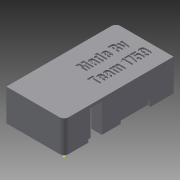
# Autodesk Inventor part: Negative Cap 545
Saved by Autodesk Inventor 2015 (Build 190159000, 159)
## iProperties
Created: 2015-01-23
Part Number: Negative Cap 545
Material: Generic
Document SubType Name: Modeling
Designer: pltwe4
Density: 1 g/cm^3
Appearance: Default
Author: pltwe4
Autodesk Inventor part; units mm, degrees
ref_plane "YZ Plane" through (0, 0, 0) normal (1, 0, 0) x (0, 1, 0)
ref_plane "XZ Plane" through (0, 0, 0) normal (0, 1, 0) x (-1, 0, 0)
ref_plane "XY Plane" through (0, 0, 0) normal (0, 0, 1) x (1, 0, 0)
sketch "Sketch1" plane through (0, 0, 0) normal (0, 1, 0) x (-1, 0, 0)
  line L0 (0, 0) -> (24.5364, 0)
  line L1 (24.5364, 0) -> (24.5364, -46.5582)
  line L2 (24.5364, -46.5582) -> (0, -46.5582)
  line L3 (0, -46.5582) -> (0, 0)
  dimension "d0" = 46.5582
  dimension "d1" = 24.5364
  constraints: 8 end point, 2 parallel, 1 horizontal, 1 perpendicular
  measures "d0" distance of L0.end L1.end
  measures "d1" distance of L1.end L2.end
extrude "Extrusion1" add sketch "Sketch1" along normal blind 13.5382
sketch "Sketch2" plane through (0, 0, 0) normal (0, -1, 0) x (1, 0, 0)
  point P0 (0, 0)
fillet "Fillet1" radius 1.905 1 edges at (-24.5364, 6.7691, -46.5582)
fillet "Fillet2" radius 1.905 1 edges at (0, 6.7691, 0)
sketch "Sketch3" plane through (0, 0, 0) normal (0, -1, 0) x (1, 0, 0)
  line L0 (-1.905, 0) -> (-24.5364, 0) projected
  arc A0 (0, -1.905) -> (-1.905, 0) centre (-1.905, -1.905) ccw projected
  line L1 (0, -46.5582) -> (0, -1.905) projected
  line L2 (-22.6314, -46.5582) -> (0, -46.5582) projected
  arc A1 (-24.5364, -44.6532) -> (-22.6314, -46.5582) centre (-22.6314, -44.6532) ccw projected
  line L3 (-24.5364, 0) -> (-24.5364, -44.6532) projected
  line L4 (-2.54, -2.54) -> (-21.9964, -2.54)
  line L5 (-21.9964, -44.0182) -> (-2.54, -44.0182)
  line L6 (0, -12.9032) -> (-4.445, -12.9032)
  line L7 (-4.445, -16.0782) -> (0, -16.0782)
  line L8 (-2.54, -44.0182) -> (-2.54, -18.6182)
  line L9 (-2.54, -10.3632) -> (-2.54, -2.54)
  line L10 (-4.445, -12.9032) -> (-4.445, -10.3632)
  line L11 (-4.445, -10.3632) -> (-2.54, -10.3632)
  line L12 (-4.445, -16.0782) -> (-4.445, -18.6182)
  line L13 (-4.445, -18.6182) -> (-2.54, -18.6182)
  line L14 (-21.9964, -10.3632) -> (-18.4404, -10.3632)
  line L15 (-18.4404, -10.3632) -> (-18.4404, -18.6182)
  line L16 (-18.4404, -18.6182) -> (-21.9964, -18.6182)
  line L17 (-21.9964, -2.54) -> (-21.9964, -10.3632)
  line L18 (-21.9964, -18.6182) -> (-21.9964, -44.0182)
  line L19 (0, -14.4907) -> (-5.2569, -14.4907) construction
  line L20 (-4.445, -11.6332) -> (-18.4404, -11.6332)
  line L21 (-4.445, -17.3482) -> (-18.4404, -17.3482)
  point P0 (0, 0)
  dimension "d7" = 2.54
  dimension "d9" = 2.54
  dimension "d11" = 3.175
  dimension "d13" = 4.445
  dimension "d14" = 2.54
  dimension "d15" = 2.54
  dimension "d16" = 2.54
  dimension "d17" = 2.54
  dimension "d20" = 2.54
  dimension "d21" = 6.096
  dimension "d22" = 2.54
  dimension "d37" = 32.0675
  constraints: 36 end point, 9 perpendicular, 7 parallel, 5 point on line, 4 horizontal, 2 collinear, 2 midpoint, 2 vertical, 1 other
  measures "d7" distance between parallel lines of L0 L4
  measures "d9" distance between parallel lines of L2 L5
  measures "d11" distance between parallel lines of L6 L7
  measures "d13" distance between parallel lines of L1 L10
  measures "d14" distance of L7.start L12.end
  measures "d15" distance of L6.end L10.end
  measures "d16" distance between parallel lines of L1 L8
  measures "d17" distance between parallel lines of L1 L9
  measures "d20" distance between parallel lines of L3 L18
  measures "d21" distance between parallel lines of L3 L15
  measures "d22" distance between parallel lines of L3 L17
  measures "d37" distance between parallel lines of L2 L19
extrude "Extrusion2" cut sketch "Sketch3" against normal blind 12.2682 contours L1 L7 L12 L21 L15 L20 L10 L6 | L20 L15 L14 L17 L4 L9 L11 L10 | L12 L13 L8 L5 L18 L16 L15 L21
sketch "Sketch4" plane through (0, 12.2682, 0) normal (0, -1, 0) x (1, 0, 0)
  line L0 (-4.3434, -23.6982) -> (-17.0434, -23.6982)
  line L1 (-17.0434, -23.6982) -> (-17.0434, -35.1282)
  line L2 (-17.0434, -35.1282) -> (-4.3434, -35.1282)
  line L3 (-4.3434, -35.1282) -> (-4.3434, -23.6982)
  line L4 (-2.54, -44.0182) -> (-21.9964, -44.0182) projected
  line L5 (-2.54, -18.6182) -> (-2.54, -44.0182) projected
  line L6 (-10.6934, -23.6982) -> (-10.6934, -35.1282) construction
  line L7 (-24.5364, 0) -> (-24.5364, -44.6532) construction
  line L8 (-22.6314, -46.5582) -> (0, -46.5582) construction
  point P0 (0, 0)
  dimension "d23" = 13.843
  dimension "d24" = 12.7
  dimension "d25" = 11.43
  dimension "d26" = 22.86
  constraints: 10 end point, 2 midpoint, 2 parallel, 1 horizontal, 1 perpendicular
  measures "d23" distance between parallel lines of L7 L6
  measures "d24" distance between parallel lines of L1 L3
  measures "d25" distance between parallel lines of L0 L2
  measures "d26" distance between parallel lines of L8 L0
extrude "Extrusion3" add sketch "Sketch4" along normal up to surface (12.2682 mm away)
sketch "Sketch5" plane through (-4.3434, 12.2682, -35.1282) normal (0, 0, -1) x (-1, 0, 0)
  line L0 (0, 0) -> (0, -12.2682) projected
  line L1 (12.7, 0) -> (12.7, -12.2682) projected
  line L2 (12.7, -12.2682) -> (0, -12.2682) projected
  arc A0 (8.2396, -6.5778) -> (4.4604, -6.5778) centre (6.35, -5.1816) ccw
  line L3 (6.35, -12.2682) -> (6.35, 0) construction
  line L4 (17.653, 0) -> (-1.8034, 0) construction
  line L5 (8.2396, -6.5778) -> (8.4707, -7.62)
  line L6 (8.4707, -7.62) -> (11.0107, -7.62)
  line L7 (11.0107, -7.62) -> (12.7, 0)
  line L8 (4.4604, -6.5778) -> (4.2293, -7.62)
  line L9 (4.2293, -7.62) -> (1.6893, -7.62)
  line L10 (1.6893, -7.62) -> (0, 0)
  point P0 (-4.3434, -12.2682)
  dimension "d29" = 7.0866
  dimension "d30" = 4.699
  dimension "d32" = 7.62
  dimension "d33" = 2.54
  dimension "d36" = 25
  constraints: 14 end point, 2 horizontal, 2 point on circle, 2 point on line, 1 centre point, 1 equal length, 1 midpoint, 1 parallel, 1 vertical, 2 other
  measures "d29" distance from line of L2 A0.centre
  measures "d30" diameter of A0
  measures "d32" distance between parallel lines of L4 L6
  measures "d33" distance of L5.end L6.end
  measures "d36" angle of L5 L8
extrude "Extrusion4" cut sketch "Sketch5" against normal up to surface (11.43 mm away)
sketch "Sketch6" plane through (0, 12.2682, 0) normal (0, -1, 0) x (1, 0, 0)
  line L0 (-4.445, -10.3632) -> (-4.445, -12.9032) projected
  line L1 (-4.445, -16.0782) -> (-4.445, -18.6182) projected
  line L2 (-18.4404, -18.6182) -> (-18.4404, -10.3632) projected
  line L3 (0, -12.9032) -> (0, -16.0782) projected
  line L4 (0, -16.0782) -> (-4.445, -16.0782) projected
  line L5 (-4.445, -12.9032) -> (0, -12.9032) projected
  line L6 (-4.445, -10.3632) -> (-18.4404, -10.3632)
  line L7 (-18.4404, -18.6182) -> (-4.445, -18.6182)
  line L8 (-1.27, -12.9032) -> (-1.27, -16.0782)
  point P0 (0, 0)
  dimension "d46" = 1.27
  constraints: 6 end point, 2 point on line, 1 horizontal, 1 parallel, 1 perpendicular
  measures "d46" distance between parallel lines of L8 L3
extrude "Extrusion5" cut sketch "Sketch6" against normal blind 0.635
sketch "Sketch7" plane through (0, 0, 0) normal (0, -1, 0) x (1, 0, 0)
  line L0 (0, -12.9032) -> (0, -1.905) projected
  line L1 (0, -1.905) -> (0, -46.5582) projected
  line L2 (0, -10.3632) -> (-0.635, -10.3632)
  line L3 (-1.27, -10.9982) -> (-1.27, -12.2682)
  arc A0 (-0.635, -10.3632) -> (-1.27, -10.9982) centre (-0.635, -10.9982) ccw
  line L4 (-1.905, -12.9032) -> (-4.445, -12.9032)
  line L5 (-4.445, -10.3632) -> (-4.445, -12.9032) projected
  arc A1 (-1.905, -12.9032) -> (-1.27, -12.2682) centre (-1.905, -12.2682) ccw
  line L6 (0, -10.3632) -> (0, -12.9032)
  line L7 (0, -12.9032) -> (-1.905, -12.9032)
  line L8 (-4.445, -12.9032) -> (0, -12.9032) projected
  point P0 (0, 0)
  point P1 (-1.27, -10.3632)
  point P2 (-1.27, -12.9032)
  dimension "d40" = 1.27
  dimension "d41" = 2.54
  dimension "d42" = 0.635
  dimension "d43" = 0.635
  constraints: 10 end point, 5 point on line, 5 tangent, 4 point on circle, 2 centre point, 2 collinear, 2 perpendicular, 1 parallel
  measures "d40" distance of L2.start point (-1.27, -10.363)
  measures "d41" distance of point (-1.27, -10.363) point (-1.27, -12.903)
  measures "d42" radius of A0
  measures "d43" radius of A1
extrude "Extrusion7" add sketch "Sketch6" against normal blind 0.635 contours L5 L3 L4 L8
extrude "Extrusion8" cut sketch "Sketch7" against normal up to surface (12.2682 mm away)
sketch "Sketch8" plane through (0, 0, -46.5582) normal (1, 0, 0) x (0, 0, -1)
  line L0 (-36.195, 0) -> (-36.195, 12.2682) projected
  line L1 (-30.48, 12.2682) -> (-36.195, 12.2682) projected
  line L2 (-30.48, 12.2682) -> (-30.48, 0) projected
  line L3 (0, 0) -> (-30.48, 0) projected
  line L4 (0, 0) -> (0, 13.5382) projected
  line L5 (-44.6532, 13.5382) -> (0, 13.5382) projected
  line L6 (-44.6532, 0) -> (-44.6532, 13.5382) projected
  line L7 (-36.195, 0) -> (-44.6532, 0) projected
  line L8 (-22.5397, 0) -> (-22.5397, 2.54)
  line L9 (-22.5397, 2.54) -> (-9.8397, 2.54)
  line L10 (-9.8397, 2.54) -> (-9.8397, 0)
  point P0 (-46.5582, 0)
  dimension "d51" = 2.54
  dimension "d52" = 12.7
  constraints: 6 end point, 2 perpendicular, 2 point on line, 1 vertical
  measures "d51" distance of L9.end L10.end
  measures "d52" distance of L8.end L9.end
extrude "Extrusion9" cut sketch "Sketch8" against normal blind 1.27 contours L8 L9 L10 L3
sketch "Sketch9" plane through (-4.3434, 12.2682, -35.1282) normal (0, 0, -1) x (-1, 0, 0)
  line L0 (12.7, 0) -> (11.0107, -7.62) projected
  line L1 (11.0107, -7.62) -> (8.4707, -7.62) projected
  line L2 (8.4707, -7.62) -> (8.2396, -6.5778) projected
  arc A0 (8.2396, -6.5778) -> (4.4604, -6.5778) centre (6.35, -5.1816) ccw projected
  line L3 (4.4604, -6.5778) -> (4.2293, -7.62) projected
  line L4 (4.2293, -7.62) -> (1.6893, -7.62) projected
  line L5 (1.6893, -7.62) -> (0, 0) projected
  line L6 (12.7, 0) -> (0, 0) projected
  line L7 (1.6893, -7.62) -> (11.0107, -7.62)
  line L8 (4.2293, -7.62) -> (1.6893, -7.62) projected
  point P0 (-4.3434, -12.2682)
  constraints: 2 end point, 1 collinear
extrude "Extrusion10" add sketch "Sketch9" along normal blind 2.54
sketch "Sketch10" plane through (0, 13.5382, 0) normal (0, 1, 0) x (1, 0, 0)
  arc A0 (-1.905, 0) -> (0, 1.905) centre (-1.905, 1.905) ccw projected
  line L0 (0, 1.905) -> (0, 46.5582) projected
  line L1 (0, 46.5582) -> (-22.6314, 46.5582) projected
  arc A1 (-22.6314, 46.5582) -> (-24.5364, 44.6532) centre (-22.6314, 44.6532) ccw projected
  line L2 (-24.5364, 44.6532) -> (-24.5364, 0) projected
  line L3 (-24.5364, 0) -> (-1.905, 0) projected
  line L4 (-17.6657, 19.1516) -> (-17.6657, 44.5516) construction
  line L5 (-17.6657, 44.5516) -> (-4.9657, 44.5516) construction
  line L6 (-4.9657, 44.5516) -> (-4.9657, 19.1516) construction
  line L7 (-4.9657, 19.1516) -> (-17.6657, 19.1516) construction
  line L8 (-17.6657, 31.8516) -> (-4.9657, 31.8516) construction
  line L9 (-24.5364, 0) -> (-24.5364, 44.6532) construction
  line L10 (-24.5364, 22.3266) -> (0, 22.3266) construction
  line L11 (-11.3157, 19.1516) -> (-11.3157, 44.5516) construction
  line L12 (-22.6314, 46.5582) -> (0, 46.5582) construction
  line L13 (-11.3157, 46.5582) -> (-11.3157, 0) construction
  line L14 (-17.6657, 25.993) -> (-13.2207, 25.993)
  line L15 (-13.2207, 25.993) -> (-13.2207, 24.9814)
  line L16 (-13.2207, 24.9814) -> (-16.222, 24.9814)
  line L17 (-16.222, 24.9814) -> (-13.2207, 24.5761)
  line L18 (-13.2207, 24.5761) -> (-13.2207, 23.8627)
  line L19 (-13.2207, 23.8627) -> (-16.155, 23.4406)
  line L20 (-16.155, 23.4406) -> (-13.2207, 23.4373)
  line L21 (-13.2207, 23.4373) -> (-13.2207, 22.4257)
  line L22 (-13.2207, 22.4257) -> (-17.6657, 22.4257)
  line L23 (-17.6657, 22.4257) -> (-17.6657, 23.923)
  spline S0 degree 2 poles (-17.6657, 23.923) (-17.2671, 23.9866) (-16.7211, 24.0603) knots 0 0 0 1 1 1
  line L24 (-16.7211, 24.0603) -> (-15.5889, 24.2244)
  line L25 (-15.5889, 24.2244) -> (-17.6657, 24.4857)
  line L26 (-17.6657, 24.4857) -> (-17.6657, 25.993)
  line L27 (-15.4549, 27.4166) -> (-15.4549, 26.3749)
  line L28 (-15.4549, 26.3749) -> (-15.6994, 26.3749)
  spline S1 degree 2 poles (-15.6994, 26.3749) (-16.1215, 26.3749) (-16.5804, 26.5692) (-16.9321, 27.1587) (-16.9321, 27.6277) knots 0 0 0 1 2 3 3 3
  spline S2 degree 2 poles (-16.9321, 27.6277) (-16.9321, 28.1904) (-16.5335, 28.7632) (-15.954, 28.8771) (-15.0496, 28.8771) knots 0 0 0 1 2 3 3 3
  line L29 (-15.0496, 28.8771) -> (-13.2207, 28.8771)
  line L30 (-13.2207, 28.8771) -> (-13.2207, 27.7985)
  line L31 (-13.2207, 27.7985) -> (-13.5456, 27.7985)
  spline S3 degree 2 poles (-13.5456, 27.7985) (-13.3513, 27.698) (-13.1537, 27.3765) (-13.1537, 27.152) knots 0 0 0 1 2 2 2
  spline S4 degree 2 poles (-13.1537, 27.152) (-13.1537, 26.8606) (-13.482, 26.3749) (-14.0347, 26.3749) knots 0 0 0 1 2 2 2
  line L32 (-14.0347, 26.3749) -> (-14.3328, 26.3749)
  spline S5 degree 2 poles (-14.3328, 26.3749) (-14.7414, 26.3749) (-15.0396, 26.6328) (-15.2372, 27.1453) knots 0 0 0 1 2 2 2
  spline S6 degree 2 poles (-15.2372, 27.1453) (-15.4516, 27.6913) (-15.599, 27.7684) (-15.8267, 27.7684) knots 0 0 0 1 2 2 2
  spline S7 degree 2 poles (-15.8267, 27.7684) (-16.1115, 27.7684) (-16.2856, 27.6846) (-16.2856, 27.5841) knots 0 0 0 1 2 2 2
  spline S8 degree 2 poles (-16.2856, 27.5841) (-16.2856, 27.4702) (-16.1416, 27.4166) (-15.8368, 27.4166) knots 0 0 0 1 2 2 2
  line L33 (-15.8368, 27.4166) -> (-15.4549, 27.4166)
  spline S9 degree 2 poles (-14.9558, 27.7684) (-14.7615, 27.5004) (-14.4969, 27.4166) (-14.249, 27.4166) knots 0 0 0 1 2 2 2
  spline S10 degree 2 poles (-14.249, 27.4166) (-13.9643, 27.4166) (-13.8002, 27.4903) (-13.8002, 27.6009) knots 0 0 0 1 2 2 2
  spline S11 degree 2 poles (-13.8002, 27.6009) (-13.8002, 27.7047) (-13.9308, 27.7684) (-14.2055, 27.7684) knots 0 0 0 1 2 2 2
  line L34 (-14.2055, 27.7684) -> (-14.9558, 27.7684)
  line L35 (-17.6657, 31.7813) -> (-13.2207, 31.7813)
  line L36 (-13.2207, 31.7813) -> (-13.2207, 30.6725)
  line L37 (-13.2207, 30.6725) -> (-13.4853, 30.6725)
  spline S12 degree 2 poles (-13.4853, 30.6725) (-13.3178, 30.5117) (-13.1537, 30.1634) (-13.1537, 29.9691) knots 0 0 0 1 2 2 2
  spline S13 degree 2 poles (-13.1537, 29.9691) (-13.1537, 29.7112) (-13.425, 29.3327) (-13.7834, 29.2255) (-14.1854, 29.2255) knots 0 0 0 1 2 3 3 3
  line L38 (-14.1854, 29.2255) -> (-15.8937, 29.2255)
  spline S14 degree 2 poles (-15.8937, 29.2255) (-16.3124, 29.2255) (-16.6642, 29.3327) (-16.9321, 29.7179) (-16.9321, 29.9825) knots 0 0 0 1 2 3 3 3
  spline S15 degree 2 poles (-16.9321, 29.9825) (-16.9321, 30.1902) (-16.7847, 30.5318) (-16.634, 30.6725) knots 0 0 0 1 2 2 2
  line L39 (-16.634, 30.6725) -> (-17.6657, 30.6725)
  line L40 (-17.6657, 30.6725) -> (-17.6657, 31.7813)
  spline S16 degree 2 poles (-15.9473, 30.6725) (-16.1483, 30.6725) (-16.2856, 30.6022) (-16.2856, 30.5017) knots 0 0 0 1 2 2 2
  spline S17 degree 2 poles (-16.2856, 30.5017) (-16.2856, 30.4045) (-16.1617, 30.3342) (-15.9473, 30.3342) knots 0 0 0 1 2 2 2
  line L41 (-15.9473, 30.3342) -> (-14.162, 30.3342)
  spline S18 degree 2 poles (-14.162, 30.3342) (-13.9409, 30.3342) (-13.8002, 30.4012) (-13.8002, 30.495) knots 0 0 0 1 2 2 2
  spline S19 degree 2 poles (-13.8002, 30.495) (-13.8002, 30.6022) (-13.9576, 30.6725) (-14.2624, 30.6725) knots 0 0 0 1 2 2 2
  line L42 (-14.2624, 30.6725) -> (-15.9473, 30.6725)
  line L43 (-14.9793, 34.6921) -> (-14.9793, 33.2551)
  line L44 (-14.9793, 33.2551) -> (-14.1921, 33.2551)
  spline S20 degree 2 poles (-14.1921, 33.2551) (-13.9442, 33.2551) (-13.8002, 33.3255) (-13.8002, 33.4293) knots 0 0 0 1 2 2 2
  spline S21 degree 2 poles (-13.8002, 33.4293) (-13.8002, 33.5566) (-13.9911, 33.6403) (-14.2624, 33.6403) knots 0 0 0 1 2 2 2
  line L45 (-14.2624, 33.6403) -> (-14.7414, 33.6403)
  line L46 (-14.7414, 33.6403) -> (-14.7414, 34.6921)
  line L47 (-14.7414, 34.6921) -> (-14.4735, 34.6921)
  spline S22 degree 2 poles (-14.4735, 34.6921) (-14.1352, 34.6921) (-13.7734, 34.6084) (-13.3614, 34.2935) (-13.1537, 33.8145) (-13.1537, 33.4494) knots 0 0 0 1 2 3 4 4 4
  spline S23 degree 2 poles (-13.1537, 33.4494) (-13.1537, 33.0977) (-13.358, 32.5617) (-13.7131, 32.2603) (-14.1385, 32.1464) (-14.5438, 32.1464) knots 0 0 0 1 2 3 4 4 4
  line L48 (-14.5438, 32.1464) -> (-15.609, 32.1464)
  spline S24 degree 2 poles (-15.609, 32.1464) (-16.0847, 32.1464) (-16.6374, 32.4043) (-16.9321, 32.9938) (-16.9321, 33.3723) knots 0 0 0 1 2 3 3 3
  spline S25 degree 2 poles (-16.9321, 33.3723) (-16.9321, 33.8413) (-16.5771, 34.4476) (-15.9942, 34.6921) (-15.4616, 34.6921) knots 0 0 0 1 2 3 3 3
  line L49 (-15.4616, 34.6921) -> (-14.9793, 34.6921)
  line L50 (-15.5722, 33.58) -> (-15.8368, 33.58)
  spline S26 degree 2 poles (-15.8368, 33.58) (-16.1215, 33.58) (-16.2856, 33.5197) (-16.2856, 33.4259) knots 0 0 0 1 2 2 2
  spline S27 degree 2 poles (-16.2856, 33.4259) (-16.2856, 33.3087) (-16.145, 33.2551) (-15.8368, 33.2551) knots 0 0 0 1 2 2 2
  line L51 (-15.8368, 33.2551) -> (-15.5722, 33.2551)
  line L52 (-15.5722, 33.2551) -> (-15.5722, 33.58)
  line L53 (-17.6657, 36.0789) -> (-17.6657, 37.2312)
  spline S28 degree 2 poles (-17.6657, 37.2312) (-17.6657, 37.7805) (-17.4949, 38.3432) (-16.9757, 38.6883) (-16.3995, 38.6883) knots 0 0 0 1 2 3 3 3
  spline S29 degree 2 poles (-16.3995, 38.6883) (-16.011, 38.6883) (-15.7028, 38.4437) (-15.6224, 38.082) knots 0 0 0 1 2 2 2
  spline S30 degree 2 poles (-15.6224, 38.082) (-15.5286, 38.4839) (-15.1099, 38.7686) (-14.6745, 38.7686) knots 0 0 0 1 2 2 2
  line L54 (-14.6745, 38.7686) -> (-14.2658, 38.7686)
  spline S31 degree 2 poles (-14.2658, 38.7686) (-13.8136, 38.7686) (-13.3815, 38.5643) (-13.2207, 38.1121) (-13.2207, 37.4154) knots 0 0 0 1 2 3 3 3
  line L55 (-13.2207, 37.4154) -> (-13.2207, 36.0789)
  line L56 (-13.2207, 36.0789) -> (-17.6657, 36.0789)
  line L57 (-15.2238, 37.2345) -> (-13.9811, 37.2345)
  spline S32 degree 2 poles (-13.9811, 37.2345) (-13.9878, 37.479) (-14.1251, 37.613) (-14.3964, 37.613) knots 0 0 0 1 2 2 2
  line L58 (-14.3964, 37.613) -> (-14.8084, 37.613)
  spline S33 degree 2 poles (-14.8084, 37.613) (-15.0965, 37.613) (-15.2171, 37.4924) (-15.2238, 37.2345) knots 0 0 0 1 2 2 2
  line L59 (-16.9053, 37.2345) -> (-15.9172, 37.2345)
  spline S34 degree 2 poles (-15.9172, 37.2345) (-15.9205, 37.3082) (-15.9205, 37.3484) knots 0 0 0 1 1 1
  spline S35 degree 2 poles (-15.9205, 37.3484) (-15.9205, 37.5192) (-16.088, 37.613) (-16.4833, 37.613) knots 0 0 0 1 2 2 2
  spline S36 degree 2 poles (-16.4833, 37.613) (-16.6909, 37.613) (-16.8584, 37.536) (-16.902, 37.412) (-16.9053, 37.2345) knots 0 0 0 1 2 3 3 3
  line L60 (-16.8651, 41.4752) -> (-14.2289, 41.157)
  spline S37 degree 2 poles (-14.2289, 41.157) (-13.6026, 41.0799) (-13.147, 40.9794) (-12.8522, 40.7449) (-12.7116, 40.3229) (-12.7116, 39.8606) knots 0 0 0 1 2 3 4 4 4
  line L61 (-12.7116, 39.8606) -> (-12.7116, 39.1874)
  line L62 (-12.7116, 39.1874) -> (-13.2944, 39.1874)
  spline S38 degree 2 poles (-13.2944, 39.1874) (-13.2944, 39.4486) (-13.348, 39.596) (-13.4384, 39.596) knots 0 0 0 1 2 2 2
  spline S39 degree 2 poles (-13.4384, 39.596) (-13.482, 39.596) (-13.8203, 39.529) knots 0 0 0 1 1 1
  line L63 (-13.8203, 39.529) -> (-16.8651, 38.9194)
  line L64 (-16.8651, 38.9194) -> (-16.8651, 39.9276)
  line L65 (-16.8651, 39.9276) -> (-14.4031, 40.2927)
  line L66 (-14.4031, 40.2927) -> (-16.8651, 40.4669)
  line L67 (-16.8651, 40.4669) -> (-16.8651, 41.4752)
  line L68 (-10.227, 22.3938) -> (-9.3359, 22.3938)
  line L69 (-9.3359, 22.3938) -> (-9.3359, 21.7072)
  line L70 (-9.3359, 21.7072) -> (-5.782, 21.7072)
  line L71 (-5.782, 21.7072) -> (-5.782, 20.5515)
  line L72 (-5.782, 20.5515) -> (-9.3359, 20.5515)
  line L73 (-9.3359, 20.5515) -> (-9.3359, 19.8682)
  line L74 (-9.3359, 19.8682) -> (-10.227, 19.8682)
  line L75 (-10.227, 19.8682) -> (-10.227, 22.3938)
  line L76 (-7.5405, 25.1372) -> (-7.5405, 23.7002)
  line L77 (-7.5405, 23.7002) -> (-6.7534, 23.7002)
  spline S40 degree 2 poles (-6.7534, 23.7002) (-6.5055, 23.7002) (-6.3614, 23.7705) (-6.3614, 23.8744) knots 0 0 0 1 2 2 2
  spline S41 degree 2 poles (-6.3614, 23.8744) (-6.3614, 24.0017) (-6.5524, 24.0854) (-6.8237, 24.0854) knots 0 0 0 1 2 2 2
  line L78 (-6.8237, 24.0854) -> (-7.3027, 24.0854)
  line L79 (-7.3027, 24.0854) -> (-7.3027, 25.1372)
  line L80 (-7.3027, 25.1372) -> (-7.0347, 25.1372)
  spline S42 degree 2 poles (-7.0347, 25.1372) (-6.6964, 25.1372) (-6.3346, 25.0535) (-5.9226, 24.7386) (-5.715, 24.2596) (-5.715, 23.8945) knots 0 0 0 1 2 3 4 4 4
  spline S43 degree 2 poles (-5.715, 23.8945) (-5.715, 23.5428) (-5.9193, 23.0068) (-6.2744, 22.7054) (-6.6998, 22.5915) (-7.1051, 22.5915) knots 0 0 0 1 2 3 4 4 4
  line L81 (-7.1051, 22.5915) -> (-8.1703, 22.5915)
  spline S44 degree 2 poles (-8.1703, 22.5915) (-8.6459, 22.5915) (-9.1986, 22.8494) (-9.4934, 23.4389) (-9.4934, 23.8174) knots 0 0 0 1 2 3 3 3
  spline S45 degree 2 poles (-9.4934, 23.8174) (-9.4934, 24.2864) (-9.1383, 24.8927) (-8.5555, 25.1372) (-8.0229, 25.1372) knots 0 0 0 1 2 3 3 3
  line L82 (-8.0229, 25.1372) -> (-7.5405, 25.1372)
  line L83 (-8.1334, 24.0251) -> (-8.398, 24.0251)
  spline S46 degree 2 poles (-8.398, 24.0251) (-8.6828, 24.0251) (-8.8469, 23.9648) (-8.8469, 23.871) knots 0 0 0 1 2 2 2
  spline S47 degree 2 poles (-8.8469, 23.871) (-8.8469, 23.7538) (-8.7062, 23.7002) (-8.398, 23.7002) knots 0 0 0 1 2 2 2
  line L84 (-8.398, 23.7002) -> (-8.1334, 23.7002)
  line L85 (-8.1334, 23.7002) -> (-8.1334, 24.0251)
  line L86 (-8.0162, 26.4905) -> (-8.0162, 25.4487)
  line L87 (-8.0162, 25.4487) -> (-8.2607, 25.4487)
  spline S48 degree 2 poles (-8.2607, 25.4487) (-8.6828, 25.4487) (-9.1417, 25.643) (-9.4934, 26.2325) (-9.4934, 26.7015) knots 0 0 0 1 2 3 3 3
  spline S49 degree 2 poles (-9.4934, 26.7015) (-9.4934, 27.2642) (-9.0948, 27.837) (-8.5153, 27.9509) (-7.6109, 27.9509) knots 0 0 0 1 2 3 3 3
  line L88 (-7.6109, 27.9509) -> (-5.782, 27.9509)
  line L89 (-5.782, 27.9509) -> (-5.782, 26.8723)
  line L90 (-5.782, 26.8723) -> (-6.1069, 26.8723)
  spline S50 degree 2 poles (-6.1069, 26.8723) (-5.9126, 26.7718) (-5.715, 26.4503) (-5.715, 26.2258) knots 0 0 0 1 2 2 2
  spline S51 degree 2 poles (-5.715, 26.2258) (-5.715, 25.9344) (-6.0432, 25.4487) (-6.5959, 25.4487) knots 0 0 0 1 2 2 2
  line L91 (-6.5959, 25.4487) -> (-6.894, 25.4487)
  spline S52 degree 2 poles (-6.894, 25.4487) (-7.3027, 25.4487) (-7.6008, 25.7066) (-7.7984, 26.2191) knots 0 0 0 1 2 2 2
  spline S53 degree 2 poles (-7.7984, 26.2191) (-8.0128, 26.7651) (-8.1602, 26.8422) (-8.388, 26.8422) knots 0 0 0 1 2 2 2
  spline S54 degree 2 poles (-8.388, 26.8422) (-8.6727, 26.8422) (-8.8469, 26.7584) (-8.8469, 26.658) knots 0 0 0 1 2 2 2
  spline S55 degree 2 poles (-8.8469, 26.658) (-8.8469, 26.5441) (-8.7029, 26.4905) (-8.398, 26.4905) knots 0 0 0 1 2 2 2
  line L92 (-8.398, 26.4905) -> (-8.0162, 26.4905)
  spline S56 degree 2 poles (-7.5171, 26.8422) (-7.3228, 26.5742) (-7.0582, 26.4905) (-6.8103, 26.4905) knots 0 0 0 1 2 2 2
  spline S57 degree 2 poles (-6.8103, 26.4905) (-6.5256, 26.4905) (-6.3614, 26.5642) (-6.3614, 26.6747) knots 0 0 0 1 2 2 2
  spline S58 degree 2 poles (-6.3614, 26.6747) (-6.3614, 26.7785) (-6.4921, 26.8422) (-6.7668, 26.8422) knots 0 0 0 1 2 2 2
  line L93 (-6.7668, 26.8422) -> (-7.5171, 26.8422)
  line L94 (-9.4264, 29.4281) -> (-9.078, 29.408)
  spline S59 degree 2 poles (-9.078, 29.408) (-9.2857, 29.5387) (-9.4934, 29.8937) (-9.4934, 30.1215) knots 0 0 0 1 2 2 2
  spline S60 degree 2 poles (-9.4934, 30.1215) (-9.4934, 30.567) (-9.078, 30.8216) knots 0 0 0 1 1 1
  spline S61 degree 2 poles (-9.078, 30.8216) (-9.2857, 30.9623) (-9.4934, 31.314) (-9.4934, 31.5284) knots 0 0 0 1 2 2 2
  spline S62 degree 2 poles (-9.4934, 31.5284) (-9.4934, 31.8097) (-9.2187, 32.1815) (-8.8201, 32.2854) (-8.3712, 32.2854) knots 0 0 0 1 2 3 3 3
  line L95 (-8.3712, 32.2854) -> (-5.782, 32.2854)
  line L96 (-5.782, 32.2854) -> (-5.782, 31.2101)
  line L97 (-5.782, 31.2101) -> (-8.1569, 31.2101)
  spline S63 degree 2 poles (-8.1569, 31.2101) (-8.6258, 31.2101) (-8.8469, 31.1465) (-8.8469, 31.0326) knots 0 0 0 1 2 2 2
  spline S64 degree 2 poles (-8.8469, 31.0326) (-8.8469, 30.912) (-8.6258, 30.845) (-8.1569, 30.845) knots 0 0 0 1 2 2 2
  line L98 (-8.1569, 30.845) -> (-5.782, 30.845)
  line L99 (-5.782, 30.845) -> (-5.782, 29.7698)
  line L100 (-5.782, 29.7698) -> (-8.0966, 29.7698)
  spline S65 degree 2 poles (-8.0966, 29.7698) (-8.6325, 29.7698) (-8.8469, 29.7162) (-8.8469, 29.599) knots 0 0 0 1 2 2 2
  spline S66 degree 2 poles (-8.8469, 29.599) (-8.8469, 29.5253) (-8.733, 29.4181) (-8.5722, 29.408) (-8.3076, 29.408) knots 0 0 0 1 2 3 3 3
  line L101 (-8.3076, 29.408) -> (-5.782, 29.408)
  line L102 (-5.782, 29.408) -> (-5.782, 28.3328)
  line L103 (-5.782, 28.3328) -> (-9.4264, 28.3328)
  line L104 (-9.4264, 28.3328) -> (-9.4264, 29.4281)
  line L105 (-10.227, 35.3704) -> (-5.782, 35.3704)
  line L106 (-5.782, 35.3704) -> (-5.782, 34.2617)
  line L107 (-5.782, 34.2617) -> (-8.1669, 34.2617)
  spline S67 degree 2 poles (-8.1669, 34.2617) (-8.6828, 34.2617) (-8.8904, 34.2114) (-8.9976, 33.9904) (-8.9976, 33.6085) knots 0 0 0 1 2 3 3 3
  line L108 (-8.9976, 33.6085) -> (-8.9976, 33.498)
  line L109 (-8.9976, 33.498) -> (-9.5168, 33.498)
  spline S68 degree 2 poles (-9.5168, 33.498) (-9.6877, 34.3019) (-10.227, 34.7206) knots 0 0 0 1 1 1
  line L110 (-10.227, 34.7206) -> (-10.227, 35.3704)
  line L111 (-10.227, 37.7587) -> (-9.2555, 37.7587)
  line L112 (-9.2555, 37.7587) -> (-5.782, 37.0519)
  line L113 (-5.782, 37.0519) -> (-5.782, 35.9466)
  line L114 (-5.782, 35.9466) -> (-9.4264, 36.7371)
  line L115 (-9.4264, 36.7371) -> (-9.4264, 35.6384)
  line L116 (-9.4264, 35.6384) -> (-10.227, 35.6384)
  line L117 (-10.227, 35.6384) -> (-10.227, 37.7587)
  line L118 (-10.227, 40.4251) -> (-9.5168, 40.4251)
  line L119 (-9.5168, 40.4251) -> (-9.5168, 39.0483)
  line L120 (-9.5168, 39.0483) -> (-8.7598, 39.0483)
  spline S69 degree 2 poles (-8.7598, 39.0483) (-9.0646, 39.3063) (-9.0646, 39.7149) knots 0 0 0 1 1 1
  spline S70 degree 2 poles (-9.0646, 39.7149) (-9.0646, 40.1738) (-8.5521, 40.6428) (-7.8219, 40.6428) knots 0 0 0 1 2 2 2
  line L121 (-7.8219, 40.6428) -> (-7.1888, 40.6428)
  spline S71 degree 2 poles (-7.1888, 40.6428) (-6.7165, 40.6428) (-6.2744, 40.5523) (-5.8992, 40.2542) (-5.6982, 39.725) (-5.6982, 39.3431) knots 0 0 0 1 2 3 4 4 4
  spline S72 degree 2 poles (-5.6982, 39.3431) (-5.6982, 38.9144) (-5.9963, 38.2612) (-6.5892, 37.9865) (-7.2089, 37.9865) knots 0 0 0 1 2 3 3 3
  line L122 (-7.2089, 37.9865) -> (-7.4501, 37.9865)
  line L123 (-7.4501, 37.9865) -> (-7.4501, 39.0952)
  line L124 (-7.4501, 39.0952) -> (-7.1721, 39.0952)
  spline S73 degree 2 poles (-7.1721, 39.0952) (-6.7433, 39.0952) (-6.3815, 39.1555) (-6.3815, 39.3364) knots 0 0 0 1 2 2 2
  spline S74 degree 2 poles (-6.3815, 39.3364) (-6.3815, 39.4168) (-6.4854, 39.5206) (-6.606, 39.5273) (-7.0716, 39.534) knots 0 0 0 1 2 3 3 3
  line L125 (-7.0716, 39.534) -> (-7.9492, 39.534)
  spline S75 degree 2 poles (-7.9492, 39.534) (-8.2004, 39.534) (-8.3813, 39.4302) (-8.3813, 39.3063) knots 0 0 0 1 2 2 2
  spline S76 degree 2 poles (-8.3813, 39.3063) (-8.3813, 39.2292) (-8.2875, 39.1254) (-8.1803, 39.0952) (-7.986, 39.0952) knots 0 0 0 1 2 3 3 3
  line L126 (-7.986, 39.0952) -> (-7.986, 37.9966)
  line L127 (-7.986, 37.9966) -> (-10.227, 38.0434)
  line L128 (-10.227, 38.0434) -> (-10.227, 40.4251)
  line L129 (-6.9644, 41.0213) -> (-6.9644, 42.13)
  spline S77 degree 2 poles (-6.9644, 42.13) (-6.6529, 42.13) (-6.4921, 42.1468) (-6.3815, 42.264) (-6.3815, 42.3679) knots 0 0 0 1 2 3 3 3
  spline S78 degree 2 poles (-6.3815, 42.3679) (-6.3815, 42.4516) (-6.4854, 42.5621) (-6.6495, 42.5755) (-6.9007, 42.5755) knots 0 0 0 1 2 3 3 3
  line L130 (-6.9007, 42.5755) -> (-7.6109, 42.5755)
  spline S79 degree 2 poles (-7.6109, 42.5755) (-7.4333, 42.4918) (-7.2525, 42.1635) (-7.2525, 41.919) knots 0 0 0 1 2 2 2
  spline S80 degree 2 poles (-7.2525, 41.919) (-7.2525, 41.6142) (-7.5807, 41.1486) (-8.043, 41.0213) (-8.4349, 41.0213) knots 0 0 0 1 2 3 3 3
  line L131 (-8.4349, 41.0213) -> (-8.7899, 41.0213)
  spline S81 degree 2 poles (-8.7899, 41.0213) (-9.2555, 41.0213) (-9.7111, 41.095) (-10.0997, 41.4032) (-10.314, 41.9458) (-10.314, 42.3076) knots 0 0 0 1 2 3 4 4 4
  spline S82 degree 2 poles (-10.314, 42.3076) (-10.314, 42.7497) (-10.0662, 43.3225) (-9.6039, 43.634) (-9.0914, 43.6843) (-8.3578, 43.6843) knots 0 0 0 1 2 3 4 4 4
  line L132 (-8.3578, 43.6843) -> (-7.7415, 43.6843)
  spline S83 degree 2 poles (-7.7415, 43.6843) (-6.9476, 43.6843) (-6.4117, 43.6407) (-5.9327, 43.3024) (-5.6949, 42.7263) (-5.6949, 42.3478) knots 0 0 0 1 2 3 4 4 4
  spline S84 degree 2 poles (-5.6949, 42.3478) (-5.6949, 41.8788) (-5.9963, 41.2826) (-6.5457, 41.0213) (-6.9644, 41.0213) knots 0 0 0 1 2 3 3 3
  spline S85 degree 2 poles (-8.3511, 42.13) (-8.0698, 42.13) (-7.9391, 42.2774) (-7.9391, 42.3545) knots 0 0 0 1 2 2 2
  spline S86 degree 2 poles (-7.9391, 42.3545) (-7.9391, 42.4684) (-8.1066, 42.5755) (-8.3511, 42.5755) knots 0 0 0 1 2 2 2
  line L133 (-8.3511, 42.5755) -> (-9.1551, 42.5755)
  spline S87 degree 2 poles (-9.1551, 42.5755) (-9.4498, 42.5755) (-9.6307, 42.475) (-9.6307, 42.3545) knots 0 0 0 1 2 2 2
  spline S88 degree 2 poles (-9.6307, 42.3545) (-9.6307, 42.2841) (-9.49, 42.13) (-9.1819, 42.13) knots 0 0 0 1 2 2 2
  line L134 (-9.1819, 42.13) -> (-8.3511, 42.13)
  point P0 (0, 0)
  dimension "d57" = 25.4
  dimension "d58" = 12.7
  dimension "d61" = 9.525
  constraints: 8 end point, 6 midpoint, 2 perpendicular, 2 point on line, 1 collinear, 2 other
  measures "d57" distance of L4.start L4.end
  measures "d58" distance of L4.end L5.end
  measures "d61" distance between parallel lines of L10 L8
extrude "Extrusion11" cut sketch "Sketch10" against normal blind 0.635 contours L14 L15 L16 L17 L18 L19 L20 L21 L22 L23 S0 L24 L25 L26 | L27 L28 S1 S2 L29 L30 L31 S3 S4 L32 S5 S6 S7 S8 L33 | L35 L36 L37 S12 S13 L38 S14 S15 L39 L40 | L43 L44 S20 S21 L45 L46 L47 S22 S23 L48 S24 S25 L49 | L53 S28 S29 S30 L54 S31 L55 L56 | L60 S37 L61 L62 S38 S39 L63 L64 L65 L66 L67 | L68 L69 L70 L71 L72 L73 L74 L75 | L76 L77 S40 S41 L78 L79 L80 S42 S43 L81 S44 S45 L82 | L86 L87 S48 S49 L88 L89 L90 S50 S51 L91 S52 S53 S54 S55 L92 | L94 S59 S60 S61 S62 L95 L96 L97 S63 S64 L98 L99 L100 S65 S66 L101 L102 L103 L104 | L105 L106 L107 S67 L108 L109 S68 L110 | L111 L112 L113 L114 L115 L116 L117 | L118 L119 L120 S69 S70 L121 S71 S72 L122 L123 L124 S73 S74 L125 S75 S76 L126 L127 L128 | L129 S77 S78 L130 S79 S80 L131 S81 S82 L132 S83 S84
equation "\"d27\" = d2"
equation "\"d34\" = d2"
equation "\"d2\" = 13.5382"
body "Solid1"
